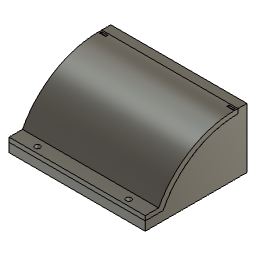
fanSocket (Autodesk Fusion 360 design; units mm, degrees)
Autodesk Fusion 360 part; units mm, degrees
sketch "Skizze1" plane through (0, 0, 0) normal (0, 1, 0) x (1, 0, 0)
  line L0 (0, 0) -> (40, 0)
  line L1 (40, 0) -> (40, -40)
  line L2 (40, -40) -> (0, -40)
  line L3 (0, -40) -> (0, 0)
  line L4 (4, -36) -> (36, -36) construction
  line L5 (36, -36) -> (36, -4) construction
  line L6 (36, -4) -> (4, -4) construction
  line L7 (4, -4) -> (4, -36) construction
  circle A0 centre (4, -36) radius 2.15
  circle A1 centre (36, -36) radius 2.15
  circle A2 centre (36, -4) radius 2.15
  circle A3 centre (4, -4) radius 2.15
  circle A4 centre (20, -20) radius 18
  dimension "d1" = 40
  dimension "d2" = 4.3
  dimension "d3" = 32
  dimension "d4" = 4
  dimension "d5" = 4
  dimension "d6" = 20
  dimension "d7" = 20
  dimension "d8" = 36
  constraint horizontal L0
  constraint vertical L1
  constraint horizontal L2
  constraint vertical L3
  constraint coincident L0.start L3.end
  constraint equal L0 L3
  constraint horizontal L4
  constraint vertical L5
  constraint horizontal L6
  constraint vertical L7
  constraint coincident L4.start L7.end
  constraint coincident L4.end L5.start
  constraint coincident L5.end L6.start
  constraint coincident L6.end L7.start
  constraint equal A0 A3
  constraint equal A0 A1
  constraint equal A1 A2
  constraint equal L4 L7
  measures "d1" distance of L0.start L2.end
  measures "d2" diameter of A0
  measures "d3" distance of L4.start L6.end
  measures "d4" vertical distance of L2.end L4.start
  measures "d5" horizontal distance of L2.end L4.start
  measures "d6" horizontal distance of L2.end A4.centre
  measures "d7" vertical distance of L1.end A4.centre
  measures "d8" diameter of A4
extrude "Extrusion1" add sketch "Skizze1" along normal blind 10 makes body 1
fillet "Abrundung1" radius 4 4 edges at (40, 5, 40) (40, 5, 0) (0, 5, 0) (0, 5, 40) on bodies 1
copy_body "Körper kopieren/einfügen1" bodies 1 makes body 2
move_body "Verschieben1" bodies 2 to x (1, 0, 0) y (0, 1, 0) z (0, 0, 1) at (41, 0, 0)
sketch "Skizze3" plane through (0, 0, 0) normal (0, 0, 1) x (1, 0, 0)
  line L0 (0, 0) -> (81, 0)
  line L1 (81, 0) -> (81, -55)
  line L2 (81, -55) -> (0, -55)
  line L3 (0, -55) -> (0, 0)
  circle A0 centre (20, -35) radius 18
  circle A1 centre (61, -35) radius 18
  circle A2 centre (40.5, -20) radius 2
  circle A3 centre (4, -51) radius 2
  circle A4 centre (77, -51) radius 2
  dimension "d15" = 20
  dimension "d16" = 20
  dimension "d17" = 36
  dimension "d18" = 40.5
  dimension "d19" = 20
  dimension "d20" = 4
  dimension "d21" = 4
  dimension "d22" = 4
  dimension "d23" = 4
  dimension "d24" = 4
  dimension "d25" = 81
  dimension "d26" = 35
  dimension "d27" = 35
  dimension "d28" = 55
  constraint horizontal L0
  constraint vertical L1
  constraint horizontal L2
  constraint vertical L3
  constraint coincident L0.start L3.end
  constraint equal A0 A1
  constraint equal A2 A3
  constraint equal A3 A4
  measures "d15" horizontal distance of L2.end A0.centre
  measures "d16" horizontal distance of L1.end A1.centre
  measures "d17" diameter of A0
  measures "d18" horizontal distance of L0.start A2.centre
  measures "d19" vertical distance of L0.start A2.centre
  measures "d20" vertical distance of L2.end A3.centre
  measures "d21" horizontal distance of L2.end A3.centre
  measures "d22" vertical distance of L1.end A4.centre
  measures "d23" horizontal distance of L1.end A4.centre
  measures "d24" diameter of A3
  measures "d25" distance of L0.start L0.end
  measures "d26" vertical distance of L0.start A0.centre
  measures "d27" vertical distance of L0.end A1.centre
  measures "d28" distance of L0.start L2.end
extrude "Extrusion2" add sketch "Skizze3" along normal blind 3 separate body makes body 3
move_body "Verschieben2" bodies 3 to x (1, 0, 0) y (0, 1, 0) z (0, 0, 1) at (0, -1, 0)
sketch "Skizze4" plane through (0, 0, 3) normal (0, 0, 1) x (-1, 0, 0)
  circle A0 centre (-40.5, 21) radius 2
  circle A1 centre (-61, 36) radius 18
  circle A2 centre (-20, 36) radius 18
  circle A3 centre (-4, 52) radius 2
  circle A4 centre (-77, 52) radius 2
  line L0 (0, 56) -> (-81, 56)
  line L1 (-81, 56) -> (-81, 1)
  line L2 (-81, 1) -> (0, 1)
  line L3 (0, 1) -> (0, 56)
  line L4 (0, 6) -> (-81, 6)
  dimension "d31" = 5
  constraint coincident L3 L4.start
  constraint coincident L1 L4.end
  constraint perpendicular L1 L4
  measures "d31" distance of L2.end L4.start
extrude "Extrusion3" add sketch "Skizze4" along normal blind 37 contours L1 L2 L3 L4 bodies 3
sketch "Skizze5" plane through (0, -6, 0) normal (0, -1, 0) x (1, 0, 0)
  line L0 (0, 3) -> (81, 3)
  line L1 (81, 3) -> (81, 40)
  line L2 (81, 40) -> (0, 40)
  line L3 (0, 40) -> (0, 3)
  line L4 (0, 20) -> (81, 20) construction
  circle A0 centre (20, 20) radius 18
  circle A1 centre (61, 20) radius 18
  line L5 (4, 36) -> (77, 36) construction
  line L6 (77, 36) -> (77, 4) construction
  line L7 (77, 4) -> (4, 4) construction
  line L8 (4, 4) -> (4, 36) construction
  circle A2 centre (4, 36) radius 2
  circle A3 centre (77, 36) radius 2
  circle A4 centre (77, 4) radius 2
  circle A5 centre (4, 4) radius 2
  line L9 (36, 36) -> (36, 4) construction
  line L10 (45, 4) -> (45, 36) construction
  circle A6 centre (36, 36) radius 2
  circle A7 centre (45, 36) radius 2
  circle A8 centre (45, 4) radius 2
  circle A9 centre (36, 4) radius 2
  dimension "d34" = 20
  dimension "d35" = 20
  dimension "d36" = 20
  dimension "d37" = 36
  dimension "d38" = 4
  dimension "d39" = 4
  dimension "d40" = 4
  dimension "d42" = 4
  dimension "d43" = 32
  dimension "d44" = 32
  dimension "d47" = 32
  constraint coincident L3 L4.start
  constraint coincident L1 L4.end
  constraint perpendicular L1 L4
  constraint coincident L4 A0.centre
  constraint coincident L4 A1.centre
  constraint equal A0 A1
  constraint perpendicular L1 L5
  constraint perpendicular L5 L8
  constraint vertical L6
  constraint horizontal L7
  constraint coincident L5.start L8.end
  constraint coincident L5.end L6.start
  constraint coincident L6.end L7.start
  constraint coincident L7.end L8.start
  constraint equal A2 A5
  constraint equal A2 A3
  constraint equal A3 A4
  constraint coincident L5 L9.start
  constraint coincident L7 L9.end
  constraint perpendicular L7 L9
  constraint coincident L7 L10.start
  constraint coincident L5 L10.end
  constraint perpendicular L5 L10
  constraint coincident L9.start A6.centre
  constraint coincident L10.end A7.centre
  constraint coincident L10.start A8.centre
  constraint coincident L9.end A9.centre
  constraint equal A8 A9
  constraint equal A7 A8
  constraint equal A6 A7
  constraint equal A2 A6
  measures "d34" distance of L2.end L4.start
  measures "d35" distance of L4.start A0.centre
  measures "d36" horizontal distance of L1.end A1.centre
  measures "d37" diameter of A0
  measures "d38" horizontal distance of L2.end L5.start
  measures "d39" vertical distance of L2.end L5.start
  measures "d40" horizontal distance of L1.end L5.end
  measures "d42" diameter of A2
  measures "d43" distance of L5.end L10.end
  measures "d44" distance of L5.start L9.start
  measures "d47" distance of L5.end L6.end
extrude "Extrusion4" cut sketch "Skizze5" against normal blind 10 contours L0 A5 | L0 A5 | L0 A0 | L0 A0 | L0 A4 | L0 A4 | L0 A9 | L0 A9 | L0 A1 | L0 A1 | L0 A8 | L0 A8 | A2 | A3 | A6 | A7 bodies 3
extrude "Extrusion18" add 1 faces at (0, -2.6667, 14.3333) along direction (-1, 0, 0) blind 5 on bodies 3 bodies 3
extrude "Extrusion19" add 1 faces at (81, -2.6667, 14.3333) along direction (1, 0, 0) blind 5 on bodies 3 bodies 3
sketch "Skizze14" plane through (0, 0, 3) normal (0, 0, 1) x (-1, 0, 0)
  circle A0 centre (-61, 36) radius 18
  circle A1 centre (-20, 36) radius 18
  circle A2 centre (-77, 52) radius 2
  circle A3 centre (-40.5, 21) radius 2
  circle A4 centre (-4, 52) radius 2
  line L0 (-75.2679, 6) -> (-66.9161, 6)
  line L1 (5, 6) -> (5, 56)
  line L2 (5, 56) -> (-86, 56)
  line L3 (-86, 56) -> (-86, 6)
  line L4 (-86, 6) -> (-78.7321, 6)
  line L5 (-25.4828, 18.8553) -> (-37.1447, 30.5172)
  line L6 (-21.8995, 18.1005) -> (-37.8995, 34.1005)
  line L7 (-17.7035, 18.1471) -> (-37.8529, 38.2965)
  line L8 (-15.3413, 18.6133) -> (-37.3867, 40.6587)
  line L9 (-12.2426, 19.7574) -> (-36.2426, 43.7574)
  line L10 (-10.4188, 20.7619) -> (-35.2381, 45.5812)
  line L11 (-7.9988, 22.5846) -> (-33.4154, 48.0012)
  line L12 (-6.5846, 23.9988) -> (-32.0012, 49.4154)
  line L13 (-4.7619, 26.4188) -> (-29.5812, 51.2381)
  line L14 (-3.7574, 28.2426) -> (-27.7574, 52.2426)
  line L15 (-2.6133, 31.3413) -> (-24.6587, 53.3867)
  line L16 (-2.1471, 33.7035) -> (-22.2965, 53.8529)
  line L17 (-2.1005, 37.8995) -> (-18.1005, 53.8995)
  line L18 (-2.8553, 41.4828) -> (-14.5172, 53.1447)
  line L19 (-66.4828, 18.8553) -> (-78.1447, 30.5172)
  line L20 (-62.8995, 18.1005) -> (-78.8995, 34.1005)
  line L21 (-58.7035, 18.1471) -> (-78.8529, 38.2965)
  line L22 (-56.3413, 18.6133) -> (-78.3867, 40.6587)
  line L23 (-53.2426, 19.7574) -> (-77.2426, 43.7574)
  line L24 (-51.4188, 20.7619) -> (-76.2381, 45.5812)
  line L25 (-48.9988, 22.5846) -> (-74.4154, 48.0012)
  line L26 (-47.5846, 23.9988) -> (-73.0012, 49.4154)
  line L27 (-45.7619, 26.4188) -> (-70.5812, 51.2381)
  line L28 (-44.7574, 28.2426) -> (-68.7574, 52.2426)
  line L29 (-43.6133, 31.3413) -> (-65.6587, 53.3867)
  line L30 (-43.1471, 33.7035) -> (-63.2965, 53.8529)
  line L31 (-59.1005, 53.8995) -> (-43.1005, 37.8995)
  line L32 (-43.8553, 41.4828) -> (-55.5172, 53.1447)
  line L33 (-78.7321, 6) -> (-75.2679, 6)
  line L34 (-66.9161, 6) -> (-55.0839, 6)
  line L35 (-55.0839, 6) -> (-46.7321, 6)
  line L36 (-46.7321, 6) -> (-43.2679, 6)
  line L37 (-43.2679, 6) -> (-37.7321, 6)
  line L38 (-37.7321, 6) -> (-34.2679, 6)
  line L39 (-34.2679, 6) -> (-25.9161, 6)
  line L40 (-25.9161, 6) -> (-14.0839, 6)
  line L41 (-14.0839, 6) -> (-5.7321, 6)
  line L42 (-5.7321, 6) -> (-2.2679, 6)
  line L43 (-2.2679, 6) -> (5, 6)
  dimension "d107" = 2
  dimension "d108" = 3
  dimension "d109" = 2
  dimension "d110" = 3
  dimension "d111" = 2
  dimension "d112" = 3
  dimension "d113" = 2
  dimension "d114" = 16
  dimension "d126" = 3
  dimension "d127" = 2
  dimension "d128" = 3
  dimension "d131" = 2
  dimension "d132" = 3
  dimension "d136" = 2
  dimension "d137" = 16
  dimension "d138" = 2
  dimension "d139" = 3
  dimension "d140" = 2
  dimension "d141" = 3
  dimension "d142" = 2
  dimension "d143" = 3
  dimension "d144" = 2
  dimension "d145" = 3
  dimension "d146" = 2
  dimension "d147" = 3
  dimension "d148" = 2
  dimension "d149" = 3
  dimension "d150" = 2
  constraint coincident A1 L5.start
  constraint coincident A1 L5.end
  constraint coincident A1 L6.start
  constraint coincident A1 L6.end
  constraint coincident A1 L7.start
  constraint coincident A1 L7.end
  constraint coincident A1 L8.start
  constraint coincident A1 L8.end
  constraint coincident A1 L9.start
  constraint coincident A1 L9.end
  constraint coincident A1 L10.start
  constraint coincident A1 L10.end
  constraint coincident A1 L11.start
  constraint coincident A1 L11.end
  constraint coincident A1 L12.start
  constraint coincident A1 L12.end
  constraint parallel L5 L6
  constraint parallel L6 L7
  constraint parallel L7 L8
  constraint parallel L8 L9
  constraint parallel L9 L10
  constraint parallel L10 L11
  constraint parallel L11 L12
  constraint coincident A1 L13.start
  constraint coincident A1 L13.end
  constraint coincident A1 L14.start
  constraint coincident A1 L14.end
  constraint coincident A1 L15.start
  constraint coincident A1 L15.end
  constraint parallel L12 L13
  constraint parallel L13 L14
  constraint parallel L14 L15
  constraint coincident A1 L16.start
  constraint coincident A1 L16.end
  constraint coincident A1 L17.start
  constraint coincident A1 L17.end
  constraint parallel L15 L16
  constraint parallel L15 L17
  constraint coincident A1 L18.start
  constraint coincident A1 L18.end
  constraint parallel L17 L18
  constraint coincident A0 L19.start
  constraint coincident A0 L19.end
  constraint coincident A0 L20.start
  constraint coincident A0 L20.end
  constraint coincident A0 L21.start
  constraint coincident A0 L21.end
  constraint coincident A0 L22.start
  constraint coincident A0 L22.end
  constraint coincident A0 L23.start
  constraint coincident A0 L23.end
  constraint coincident A0 L24.start
  constraint coincident A0 L24.end
  constraint coincident A0 L25.start
  constraint coincident A0 L25.end
  constraint coincident A0 L26.start
  constraint coincident A0 L26.end
  constraint coincident A0 L27.start
  constraint coincident A0 L27.end
  constraint coincident A0 L28.start
  constraint coincident A0 L28.end
  constraint coincident A0 L29.start
  constraint coincident A0 L29.end
  constraint coincident A0 L30.start
  constraint coincident A0 L30.end
  constraint coincident A0 L31.start
  constraint coincident A0 L31.end
  constraint coincident A0 L32.start
  constraint coincident A0 L32.end
  constraint parallel L19 L20
  constraint parallel L20 L21
  constraint parallel L21 L22
  constraint parallel L22 L23
  constraint parallel L23 L24
  constraint parallel L24 L25
  constraint parallel L25 L26
  constraint parallel L26 L27
  constraint parallel L27 L28
  constraint parallel L28 L29
  constraint parallel L29 L30
  constraint parallel L30 L31
  constraint parallel L31 L32
  measures "d107" distance of L5 L6
  measures "d108" distance of L6 L7
  measures "d109" distance of L7 L8
  measures "d110" distance of L8 L9
  measures "d111" distance of L9 L10
  measures "d112" distance of L10 L11
  measures "d113" distance of L11 L12
  measures "d114" distance of A1.centre L5
  measures "d126" distance of L12 L13
  measures "d127" distance of L13 L14
  measures "d128" distance of L14 L15
  measures "d131" distance of L15 L16
  measures "d132" distance of L16 L17
  measures "d136" distance of L17 L18
  measures "d137" distance of A0.centre L19
  measures "d138" distance of L19 L20
  measures "d139" distance of L20 L21
  measures "d140" distance of L21 L22
  measures "d141" distance of L22 L23
  measures "d142" distance of L23 L24
  measures "d143" distance of L24 L25
  measures "d144" distance of L25 L26
  measures "d145" distance of L26 L27
  measures "d146" distance of L27 L28
  measures "d147" distance of L28 L29
  measures "d148" distance of L29 L30
  measures "d149" distance of L30 L31
  measures "d150" distance of L31 L32
extrude "Extrusion25" add sketch "Skizze14" against normal blind 3 contours A0 L31 L32 | A0 L29 L30 | A0 L27 L28 | A0 L25 L26 | A0 L23 L24 | A0 L21 L22 | A0 L19 L20 | A1 L17 L18 | A1 L15 L16 | A1 L13 L14 | A1 L11 L12 | A1 L9 L10 | A1 L7 L8 | A1 L5 L6 bodies 3
extrude "Extrusion28" add 1 faces at (25.3333, -56, 1) along direction (0, -1, 0) blind 12 on bodies 3 bodies 3
sketch "Skizze19" plane through (0, 0, 3) normal (0, 0, 1) x (-1, 0, 0)
  circle A0 centre (-40.5, 21) radius 2
  circle A1 centre (-4, 52) radius 2
  circle A2 centre (-77, 52) radius 2
  line L0 (-78.1447, 30.5172) -> (-66.4828, 18.8553)
  arc A3 (-78.1447, 30.5172) -> (-66.4828, 18.8553) centre (-61, 36) ccw
  line L1 (-37.1447, 30.5172) -> (-25.4828, 18.8553)
  arc A4 (-37.1447, 30.5172) -> (-25.4828, 18.8553) centre (-20, 36) ccw
  line L2 (-74.4154, 48.0012) -> (-48.9988, 22.5846)
  arc A5 (-51.4188, 20.7619) -> (-48.9988, 22.5846) centre (-61, 36) ccw
  line L3 (-51.4188, 20.7619) -> (-76.2381, 45.5812)
  arc A6 (-74.4154, 48.0012) -> (-76.2381, 45.5812) centre (-61, 36) ccw
  arc A7 (-43.8553, 41.4828) -> (-55.5172, 53.1447) centre (-61, 36) ccw
  line L4 (-43.8553, 41.4828) -> (-55.5172, 53.1447)
  line L5 (-29.5812, 51.2381) -> (-4.7619, 26.4188)
  arc A8 (-6.5846, 23.9988) -> (-4.7619, 26.4188) centre (-20, 36) ccw
  line L6 (-6.5846, 23.9988) -> (-32.0012, 49.4154)
  arc A9 (-29.5812, 51.2381) -> (-32.0012, 49.4154) centre (-20, 36) ccw
  line L7 (-37.8529, 38.2965) -> (-17.7035, 18.1471)
  arc A10 (-21.8995, 18.1005) -> (-17.7035, 18.1471) centre (-20, 36) ccw
  line L8 (-21.8995, 18.1005) -> (-37.8995, 34.1005)
  arc A11 (-37.8529, 38.2965) -> (-37.8995, 34.1005) centre (-20, 36) ccw
  line L9 (-24.6587, 53.3867) -> (-2.6133, 31.3413)
  arc A12 (-3.7574, 28.2426) -> (-2.6133, 31.3413) centre (-20, 36) ccw
  line L10 (-3.7574, 28.2426) -> (-27.7574, 52.2426)
  arc A13 (-24.6587, 53.3867) -> (-27.7574, 52.2426) centre (-20, 36) ccw
  arc A14 (-59.1005, 53.8995) -> (-63.2965, 53.8529) centre (-61, 36) ccw
  line L11 (-59.1005, 53.8995) -> (-43.1005, 37.8995)
  arc A15 (-43.1471, 33.7035) -> (-43.1005, 37.8995) centre (-61, 36) ccw
  line L12 (-43.1471, 33.7035) -> (-63.2965, 53.8529)
  arc A16 (-77.2426, 43.7574) -> (-78.3867, 40.6587) centre (-61, 36) ccw
  line L13 (-77.2426, 43.7574) -> (-53.2426, 19.7574)
  arc A17 (-56.3413, 18.6133) -> (-53.2426, 19.7574) centre (-61, 36) ccw
  line L14 (-56.3413, 18.6133) -> (-78.3867, 40.6587)
  line L15 (-70.5812, 51.2381) -> (-45.7619, 26.4188)
  arc A18 (-47.5846, 23.9988) -> (-45.7619, 26.4188) centre (-61, 36) ccw
  line L16 (-47.5846, 23.9988) -> (-73.0012, 49.4154)
  arc A19 (-70.5812, 51.2381) -> (-73.0012, 49.4154) centre (-61, 36) ccw
  arc A20 (-2.8553, 41.4828) -> (-14.5172, 53.1447) centre (-20, 36) ccw
  line L17 (-2.8553, 41.4828) -> (-14.5172, 53.1447)
  arc A21 (-33.4154, 48.0012) -> (-35.2381, 45.5812) centre (-20, 36) ccw
  line L18 (-33.4154, 48.0012) -> (-7.9988, 22.5846)
  arc A22 (-10.4188, 20.7619) -> (-7.9988, 22.5846) centre (-20, 36) ccw
  line L19 (-10.4188, 20.7619) -> (-35.2381, 45.5812)
  arc A23 (-36.2426, 43.7574) -> (-37.3867, 40.6587) centre (-20, 36) ccw
  line L20 (-36.2426, 43.7574) -> (-12.2426, 19.7574)
  arc A24 (-15.3413, 18.6133) -> (-12.2426, 19.7574) centre (-20, 36) ccw
  line L21 (-15.3413, 18.6133) -> (-37.3867, 40.6587)
  arc A25 (-18.1005, 53.8995) -> (-22.2965, 53.8529) centre (-20, 36) ccw
  line L22 (-18.1005, 53.8995) -> (-2.1005, 37.8995)
  arc A26 (-2.1471, 33.7035) -> (-2.1005, 37.8995) centre (-20, 36) ccw
  line L23 (-2.1471, 33.7035) -> (-22.2965, 53.8529)
  arc A27 (-65.6587, 53.3867) -> (-68.7574, 52.2426) centre (-61, 36) ccw
  line L24 (-65.6587, 53.3867) -> (-43.6133, 31.3413)
  arc A28 (-44.7574, 28.2426) -> (-43.6133, 31.3413) centre (-61, 36) ccw
  line L25 (-44.7574, 28.2426) -> (-68.7574, 52.2426)
  arc A29 (-78.8529, 38.2965) -> (-78.8995, 34.1005) centre (-61, 36) ccw
  line L26 (-78.8529, 38.2965) -> (-58.7035, 18.1471)
  arc A30 (-62.8995, 18.1005) -> (-58.7035, 18.1471) centre (-61, 36) ccw
  line L27 (-62.8995, 18.1005) -> (-78.8995, 34.1005)
  line L28 (-86, 6) -> (-78.7321, 6)
  line L29 (5, 6) -> (5, 68)
  line L30 (5, 68) -> (-86, 68)
  line L31 (-86, 68) -> (-86, 6)
  line L32 (5, 64) -> (-86, 64) construction
  circle A31 centre (-10, 64) radius 2
  circle A32 centre (-71, 64) radius 2
  line L33 (-78.7321, 6) -> (-75.2679, 6)
  line L34 (-75.2679, 6) -> (-66.9161, 6)
  line L35 (-66.9161, 6) -> (-55.0839, 6)
  line L36 (-55.0839, 6) -> (-46.7321, 6)
  line L37 (-46.7321, 6) -> (-43.2679, 6)
  line L38 (-43.2679, 6) -> (-37.7321, 6)
  line L39 (-37.7321, 6) -> (-34.2679, 6)
  line L40 (-34.2679, 6) -> (-25.9161, 6)
  line L41 (-25.9161, 6) -> (-14.0839, 6)
  line L42 (-14.0839, 6) -> (-5.7321, 6)
  line L43 (-5.7321, 6) -> (-2.2679, 6)
  line L44 (-2.2679, 6) -> (5, 6)
  dimension "d163" = 4
  dimension "d164" = 15
  dimension "d165" = 15
  dimension "d176" = 4
  dimension "d177" = 91
  constraint coincident L32 A31.centre
  constraint coincident L32 A32.centre
  constraint equal A31 A32
  constraint horizontal L32
  constraint coincident L29 L32.start
  measures "d163" diameter of A31
  measures "d164" distance of L32.start A31.centre
  measures "d165" distance of L32.end A32.centre
  measures "d176" distance of L29.end L32.start
  measures "d177" distance of L32.start L32.end
extrude "Extrusion29" cut sketch "Skizze19" against normal blind 5 contours A31 | A32 bodies 3
sketch "Skizze21" plane through (0, 0, 3) normal (0, 0, 1) x (-1, 0, 0)
  circle A0 centre (-40.5, 21) radius 2
  circle A1 centre (-4, 52) radius 2
  circle A2 centre (-77, 52) radius 2
  line L0 (-78.1447, 30.5172) -> (-66.4828, 18.8553)
  arc A3 (-78.1447, 30.5172) -> (-66.4828, 18.8553) centre (-61, 36) ccw
  line L1 (-37.1447, 30.5172) -> (-25.4828, 18.8553)
  arc A4 (-37.1447, 30.5172) -> (-25.4828, 18.8553) centre (-20, 36) ccw
  line L2 (-74.4154, 48.0012) -> (-48.9988, 22.5846)
  arc A5 (-51.4188, 20.7619) -> (-48.9988, 22.5846) centre (-61, 36) ccw
  line L3 (-51.4188, 20.7619) -> (-76.2381, 45.5812)
  arc A6 (-74.4154, 48.0012) -> (-76.2381, 45.5812) centre (-61, 36) ccw
  arc A7 (-43.8553, 41.4828) -> (-55.5172, 53.1447) centre (-61, 36) ccw
  line L4 (-43.8553, 41.4828) -> (-55.5172, 53.1447)
  line L5 (-29.5812, 51.2381) -> (-4.7619, 26.4188)
  arc A8 (-6.5846, 23.9988) -> (-4.7619, 26.4188) centre (-20, 36) ccw
  line L6 (-6.5846, 23.9988) -> (-32.0012, 49.4154)
  arc A9 (-29.5812, 51.2381) -> (-32.0012, 49.4154) centre (-20, 36) ccw
  line L7 (-37.8529, 38.2965) -> (-17.7035, 18.1471)
  arc A10 (-21.8995, 18.1005) -> (-17.7035, 18.1471) centre (-20, 36) ccw
  line L8 (-21.8995, 18.1005) -> (-37.8995, 34.1005)
  arc A11 (-37.8529, 38.2965) -> (-37.8995, 34.1005) centre (-20, 36) ccw
  line L9 (-24.6587, 53.3867) -> (-2.6133, 31.3413)
  arc A12 (-3.7574, 28.2426) -> (-2.6133, 31.3413) centre (-20, 36) ccw
  line L10 (-3.7574, 28.2426) -> (-27.7574, 52.2426)
  arc A13 (-24.6587, 53.3867) -> (-27.7574, 52.2426) centre (-20, 36) ccw
  arc A14 (-59.1005, 53.8995) -> (-63.2965, 53.8529) centre (-61, 36) ccw
  line L11 (-59.1005, 53.8995) -> (-43.1005, 37.8995)
  arc A15 (-43.1471, 33.7035) -> (-43.1005, 37.8995) centre (-61, 36) ccw
  line L12 (-43.1471, 33.7035) -> (-63.2965, 53.8529)
  arc A16 (-77.2426, 43.7574) -> (-78.3867, 40.6587) centre (-61, 36) ccw
  line L13 (-77.2426, 43.7574) -> (-53.2426, 19.7574)
  arc A17 (-56.3413, 18.6133) -> (-53.2426, 19.7574) centre (-61, 36) ccw
  line L14 (-56.3413, 18.6133) -> (-78.3867, 40.6587)
  line L15 (-70.5812, 51.2381) -> (-45.7619, 26.4188)
  arc A18 (-47.5846, 23.9988) -> (-45.7619, 26.4188) centre (-61, 36) ccw
  line L16 (-47.5846, 23.9988) -> (-73.0012, 49.4154)
  arc A19 (-70.5812, 51.2381) -> (-73.0012, 49.4154) centre (-61, 36) ccw
  arc A20 (-2.8553, 41.4828) -> (-14.5172, 53.1447) centre (-20, 36) ccw
  line L17 (-2.8553, 41.4828) -> (-14.5172, 53.1447)
  arc A21 (-33.4154, 48.0012) -> (-35.2381, 45.5812) centre (-20, 36) ccw
  line L18 (-33.4154, 48.0012) -> (-7.9988, 22.5846)
  arc A22 (-10.4188, 20.7619) -> (-7.9988, 22.5846) centre (-20, 36) ccw
  line L19 (-10.4188, 20.7619) -> (-35.2381, 45.5812)
  arc A23 (-36.2426, 43.7574) -> (-37.3867, 40.6587) centre (-20, 36) ccw
  line L20 (-36.2426, 43.7574) -> (-12.2426, 19.7574)
  arc A24 (-15.3413, 18.6133) -> (-12.2426, 19.7574) centre (-20, 36) ccw
  line L21 (-15.3413, 18.6133) -> (-37.3867, 40.6587)
  arc A25 (-18.1005, 53.8995) -> (-22.2965, 53.8529) centre (-20, 36) ccw
  line L22 (-18.1005, 53.8995) -> (-2.1005, 37.8995)
  arc A26 (-2.1471, 33.7035) -> (-2.1005, 37.8995) centre (-20, 36) ccw
  line L23 (-2.1471, 33.7035) -> (-22.2965, 53.8529)
  arc A27 (-65.6587, 53.3867) -> (-68.7574, 52.2426) centre (-61, 36) ccw
  line L24 (-65.6587, 53.3867) -> (-43.6133, 31.3413)
  arc A28 (-44.7574, 28.2426) -> (-43.6133, 31.3413) centre (-61, 36) ccw
  line L25 (-44.7574, 28.2426) -> (-68.7574, 52.2426)
  arc A29 (-78.8529, 38.2965) -> (-78.8995, 34.1005) centre (-61, 36) ccw
  line L26 (-78.8529, 38.2965) -> (-58.7035, 18.1471)
  arc A30 (-62.8995, 18.1005) -> (-58.7035, 18.1471) centre (-61, 36) ccw
  line L27 (-62.8995, 18.1005) -> (-78.8995, 34.1005)
  line L28 (-86, 6) -> (-78.7321, 6)
  line L29 (5, 6) -> (5, 68)
  line L30 (5, 68) -> (-86, 68)
  line L31 (-86, 68) -> (-86, 6)
  line L32 (5, 56) -> (-86, 56)
  circle A31 centre (-71, 64) radius 2
  circle A32 centre (-10, 64) radius 2
  line L33 (-78.7321, 6) -> (-75.2679, 6)
  line L34 (-75.2679, 6) -> (-66.9161, 6)
  line L35 (-66.9161, 6) -> (-55.0839, 6)
  line L36 (-55.0839, 6) -> (-46.7321, 6)
  line L37 (-46.7321, 6) -> (-43.2679, 6)
  line L38 (-43.2679, 6) -> (-37.7321, 6)
  line L39 (-37.7321, 6) -> (-34.2679, 6)
  line L40 (-34.2679, 6) -> (-25.9161, 6)
  line L41 (-25.9161, 6) -> (-14.0839, 6)
  line L42 (-14.0839, 6) -> (-5.7321, 6)
  line L43 (-5.7321, 6) -> (-2.2679, 6)
  line L44 (-2.2679, 6) -> (5, 6)
  dimension "d172" = 12
  constraint coincident L29 L32.start
  constraint coincident L31 L32.end
  constraint perpendicular L31 L32
  measures "d172" distance of L29.end L32.start
extrude "Extrusion32" add sketch "Skizze21" along normal blind 3 contours L29 L30 L31 L32 bodies 3
sketch "Skizze22" plane through (-5, 0, 0) normal (-1, 0, 0) x (0, -1, 0)
  line L0 (1, 0) -> (68, 0)
  line L1 (68, 0) -> (68, 6)
  line L2 (68, 6) -> (56, 6)
  line L3 (56, 6) -> (56, 3)
  line L4 (56, 3) -> (6, 3)
  line L5 (6, 3) -> (6, 40)
  line L6 (6, 40) -> (1, 40)
  line L7 (1, 40) -> (1, 0)
  arc A0 (56, 6) -> (6, 37) centre (6, -18.8226) ccw
  line L8 (6, 37) -> (1, 37)
  dimension "d182" = 3
  constraint coincident L2.end L3.start
  constraint coincident L5 A0.end
  constraint coincident L7 L8.end
  constraint perpendicular L7 L8
  constraint tangent A0 L8
  measures "d182" distance of L5.end A0.end
extrude "Extrusion34" add sketch "Skizze22" against normal blind 3 contours L3 L4 L5 A0 bodies 3
sketch "Skizze23" plane through (86, 0, 0) normal (1, 0, 0) x (0, 1, 0)
  line L0 (-68, 0) -> (-1, 0)
  line L1 (-1, 0) -> (-1, 40)
  line L2 (-1, 40) -> (-6, 40)
  line L3 (-6, 40) -> (-6, 3)
  line L4 (-6, 3) -> (-56, 3)
  line L5 (-56, 3) -> (-56, 6)
  line L6 (-56, 6) -> (-68, 6)
  line L7 (-68, 6) -> (-68, 0)
  arc A0 (-6, 37) -> (-56, 6) centre (-6, -18.8226) ccw
  line L8 (-6, 37) -> (-1, 37)
  dimension "d185" = 3
  constraint coincident L5.end L6.start
  constraint coincident L3 A0.start
  constraint coincident L1 L8.end
  constraint tangent A0 L8
  constraint horizontal L8
  measures "d185" distance of L2.end A0.start
extrude "Extrusion35" add sketch "Skizze23" against normal blind 3 contours L3 L4 L5 A0 bodies 3
sketch "Skizze24" plane through (0, 0, 0) normal (1, 0, 0) x (0, 1, 0)
  arc A0 (-6, 37) -> (-56, 6) centre (-6.2378, -18.439) ccw
  line L0 (-6, 37) -> (-6, 40)
  line L1 (-56, 6) -> (-59, 6)
  line L2 (-59, 6) -> (-59, 9) construction
  arc A1 (-6, 40) -> (-59, 9) centre (-7.9795, -17.4222) ccw
  line L3 (-59, 9) -> (-68, 9)
  line L4 (-68, 9) -> (-68, 6)
  line L5 (-68, 6) -> (-59, 6)
  dimension "d188" = 3
  dimension "d189" = 9
  dimension "d190" = 3
  constraint vertical L0
  constraint horizontal L1
  constraint perpendicular L1 L2
  constraint tangent A0 A1
  constraint perpendicular L2 L3
  constraint perpendicular L3 L4
  constraint perpendicular L2 L5
  measures "d188" distance of A0.end L1.end
  measures "d189" distance of L2.end L3.end
  measures "d190" distance of L3.end L4.end
extrude "Extrusion36" add sketch "Skizze24" along normal blind 91 separate body makes body 4
move_body "Verschieben4" bodies 4 to x (1, 0, 0) y (0, 1, 0) z (0, 0, 1) at (-5, 0, 0)
sketch "Skizze26" plane through (0, 0, 6) normal (0, 0, -1) x (1, 0, 0)
  line L0 (-5, 68) -> (-5, 59)
  line L1 (-5, 59) -> (86, 59)
  line L2 (86, 59) -> (86, 68)
  line L3 (86, 68) -> (-5, 68)
  circle A0 centre (10, 64) radius 1.75
  circle A1 centre (71, 64) radius 1.75
  dimension "d193" = 3.5
  dimension "d194" = 3.5
  measures "d193" diameter of A1
  measures "d194" diameter of A0
extrude "Extrusion37" cut sketch "Skizze26" against normal blind 10 contours A0 | A1 bodies 4
sketch "Skizze30" plane through (0, -6, 0) normal (0, -1, 0) x (1, 0, 0)
  line L0 (83, 37) -> (86, 37)
  line L1 (86, 37) -> (86, 40)
  line L2 (86, 40) -> (-5, 40)
  line L3 (-5, 40) -> (-5, 37)
  line L4 (-5, 37) -> (-2, 37)
  line L5 (-2, 37) -> (-2, 3)
  line L6 (-2, 3) -> (2.2679, 3)
  line L7 (78.7321, 3) -> (83, 3)
  line L8 (83, 3) -> (83, 37)
  circle A0 centre (77, 36) radius 2
  circle A1 centre (4, 36) radius 2
  circle A2 centre (36, 36) radius 2
  circle A3 centre (45, 36) radius 2
  arc A4 (5.7321, 3) -> (2.2679, 3) centre (4, 4) ccw
  line L9 (5.7321, 3) -> (14.0839, 3)
  arc A5 (25.9161, 3) -> (14.0839, 3) centre (20, 20) ccw
  line L10 (25.9161, 3) -> (34.2679, 3)
  arc A6 (37.7321, 3) -> (34.2679, 3) centre (36, 4) ccw
  line L11 (37.7321, 3) -> (43.2679, 3)
  arc A7 (46.7321, 3) -> (43.2679, 3) centre (45, 4) ccw
  line L12 (46.7321, 3) -> (55.0839, 3)
  arc A8 (66.9161, 3) -> (55.0839, 3) centre (61, 20) ccw
  line L13 (66.9161, 3) -> (75.2679, 3)
  arc A9 (78.7321, 3) -> (75.2679, 3) centre (77, 4) ccw
  line L14 (-4, 38.5) -> (0, 38.5)
  line L15 (0, 38.5) -> (0, 37)
  line L16 (0, 37) -> (-4, 37)
  line L17 (-4, 37) -> (-4, 38.5)
  line L18 (85, 38.5) -> (81, 38.5)
  line L19 (81, 38.5) -> (81, 37)
  line L20 (81, 37) -> (85, 37)
  line L21 (85, 37) -> (85, 38.5)
  dimension "d237" = 4
  dimension "d238" = 1.5
  dimension "d239" = 1.5
  dimension "d240" = 1
  dimension "d241" = 4
  dimension "d242" = 1.5
  dimension "d243" = 1
  dimension "d244" = 1.5
  constraint horizontal L14
  constraint vertical L15
  constraint horizontal L16
  constraint vertical L17
  constraint horizontal L18
  constraint vertical L19
  constraint horizontal L20
  constraint vertical L21
  measures "d237" distance of L14.start L14.end
  measures "d238" vertical distance of L2.end L14.start
  measures "d239" distance of L14.start L16.end
  measures "d240" horizontal distance of L2.end L14.start
  measures "d241" distance of L18.start L18.end
  measures "d242" vertical distance of L1.end L18.start
  measures "d243" horizontal distance of L1.end L18.start
  measures "d244" distance of L18.start L20.end
extrude "Extrusion41" add 1 faces at (83.6667, -1, 20) along direction (0, 1, 0) blind 1 on bodies 3 bodies 3
sketch "Skizze31" plane through (0, 0, 3) normal (0, 0, 1) x (-1, 0, 0)
  line L0 (-83, 56) -> (-83, 6)
  line L1 (-83, 6) -> (-78.7321, 6)
  line L2 (-78.7321, 6) -> (-75.2679, 6)
  line L3 (-75.2679, 6) -> (-66.9161, 6)
  line L4 (-66.9161, 6) -> (-55.0839, 6)
  line L5 (-55.0839, 6) -> (-46.7321, 6)
  line L6 (-46.7321, 6) -> (-43.2679, 6)
  line L7 (-43.2679, 6) -> (-37.7321, 6)
  line L8 (-37.7321, 6) -> (-34.2679, 6)
  line L9 (-34.2679, 6) -> (-25.9161, 6)
  line L10 (-25.9161, 6) -> (-14.0839, 6)
  line L11 (-14.0839, 6) -> (-5.7321, 6)
  line L12 (-5.7321, 6) -> (-2.2679, 6)
  line L13 (-2.2679, 6) -> (2, 6)
  line L14 (2, 6) -> (2, 56)
  line L15 (2, 56) -> (-83, 56)
  arc A0 (-78.8529, 38.2965) -> (-78.8995, 34.1005) centre (-61, 36) ccw
  line L16 (-78.8529, 38.2965) -> (-58.7035, 18.1471)
  arc A1 (-62.8995, 18.1005) -> (-58.7035, 18.1471) centre (-61, 36) ccw
  line L17 (-62.8995, 18.1005) -> (-78.8995, 34.1005)
  arc A2 (-65.6587, 53.3867) -> (-68.7574, 52.2426) centre (-61, 36) ccw
  line L18 (-65.6587, 53.3867) -> (-43.6133, 31.3413)
  arc A3 (-44.7574, 28.2426) -> (-43.6133, 31.3413) centre (-61, 36) ccw
  line L19 (-44.7574, 28.2426) -> (-68.7574, 52.2426)
  arc A4 (-18.1005, 53.8995) -> (-22.2965, 53.8529) centre (-20, 36) ccw
  line L20 (-18.1005, 53.8995) -> (-2.1005, 37.8995)
  arc A5 (-2.1471, 33.7035) -> (-2.1005, 37.8995) centre (-20, 36) ccw
  line L21 (-2.1471, 33.7035) -> (-22.2965, 53.8529)
  arc A6 (-36.2426, 43.7574) -> (-37.3867, 40.6587) centre (-20, 36) ccw
  line L22 (-36.2426, 43.7574) -> (-12.2426, 19.7574)
  arc A7 (-15.3413, 18.6133) -> (-12.2426, 19.7574) centre (-20, 36) ccw
  line L23 (-15.3413, 18.6133) -> (-37.3867, 40.6587)
  arc A8 (-33.4154, 48.0012) -> (-35.2381, 45.5812) centre (-20, 36) ccw
  line L24 (-33.4154, 48.0012) -> (-7.9988, 22.5846)
  arc A9 (-10.4188, 20.7619) -> (-7.9988, 22.5846) centre (-20, 36) ccw
  line L25 (-10.4188, 20.7619) -> (-35.2381, 45.5812)
  arc A10 (-2.8553, 41.4828) -> (-14.5172, 53.1447) centre (-20, 36) ccw
  line L26 (-2.8553, 41.4828) -> (-14.5172, 53.1447)
  line L27 (-70.5812, 51.2381) -> (-45.7619, 26.4188)
  arc A11 (-47.5846, 23.9988) -> (-45.7619, 26.4188) centre (-61, 36) ccw
  line L28 (-47.5846, 23.9988) -> (-73.0012, 49.4154)
  arc A12 (-70.5812, 51.2381) -> (-73.0012, 49.4154) centre (-61, 36) ccw
  arc A13 (-77.2426, 43.7574) -> (-78.3867, 40.6587) centre (-61, 36) ccw
  line L29 (-77.2426, 43.7574) -> (-53.2426, 19.7574)
  arc A14 (-56.3413, 18.6133) -> (-53.2426, 19.7574) centre (-61, 36) ccw
  line L30 (-56.3413, 18.6133) -> (-78.3867, 40.6587)
  arc A15 (-59.1005, 53.8995) -> (-63.2965, 53.8529) centre (-61, 36) ccw
  line L31 (-59.1005, 53.8995) -> (-43.1005, 37.8995)
  arc A16 (-43.1471, 33.7035) -> (-43.1005, 37.8995) centre (-61, 36) ccw
  line L32 (-43.1471, 33.7035) -> (-63.2965, 53.8529)
  line L33 (-24.6587, 53.3867) -> (-2.6133, 31.3413)
  arc A17 (-3.7574, 28.2426) -> (-2.6133, 31.3413) centre (-20, 36) ccw
  line L34 (-3.7574, 28.2426) -> (-27.7574, 52.2426)
  arc A18 (-24.6587, 53.3867) -> (-27.7574, 52.2426) centre (-20, 36) ccw
  line L35 (-37.8529, 38.2965) -> (-17.7035, 18.1471)
  arc A19 (-21.8995, 18.1005) -> (-17.7035, 18.1471) centre (-20, 36) ccw
  line L36 (-21.8995, 18.1005) -> (-37.8995, 34.1005)
  arc A20 (-37.8529, 38.2965) -> (-37.8995, 34.1005) centre (-20, 36) ccw
  line L37 (-29.5812, 51.2381) -> (-4.7619, 26.4188)
  arc A21 (-6.5846, 23.9988) -> (-4.7619, 26.4188) centre (-20, 36) ccw
  line L38 (-6.5846, 23.9988) -> (-32.0012, 49.4154)
  arc A22 (-29.5812, 51.2381) -> (-32.0012, 49.4154) centre (-20, 36) ccw
  arc A23 (-43.8553, 41.4828) -> (-55.5172, 53.1447) centre (-61, 36) ccw
  line L39 (-43.8553, 41.4828) -> (-55.5172, 53.1447)
  line L40 (-74.4154, 48.0012) -> (-48.9988, 22.5846)
  arc A24 (-51.4188, 20.7619) -> (-48.9988, 22.5846) centre (-61, 36) ccw
  line L41 (-51.4188, 20.7619) -> (-76.2381, 45.5812)
  arc A25 (-74.4154, 48.0012) -> (-76.2381, 45.5812) centre (-61, 36) ccw
  circle A26 centre (-77, 52) radius 2
  circle A27 centre (-4, 52) radius 2
  circle A28 centre (-40.5, 21) radius 2
  line L42 (-37.1447, 30.5172) -> (-25.4828, 18.8553)
  arc A29 (-37.1447, 30.5172) -> (-25.4828, 18.8553) centre (-20, 36) ccw
  line L43 (-78.1447, 30.5172) -> (-66.4828, 18.8553)
  arc A30 (-78.1447, 30.5172) -> (-66.4828, 18.8553) centre (-61, 36) ccw
  circle A31 centre (-40.5, 21) radius 5
  line L44 (2, 47) -> (-5.7522, 47)
  line L45 (-9, 56) -> (-9, 50.2478)
  line L46 (-74.4154, 48.0012) -> (-73.0012, 49.4154)
  line L47 (-75.2478, 47) -> (-83, 47)
  line L48 (-72, 50.2478) -> (-72, 56)
  dimension "d221" = 10
  dimension "d222" = 5
  dimension "d223" = 5
  dimension "d225" = 5
  dimension "d226" = 5
  constraint concentric A28 A31
  constraint coincident L14 L44.start
  constraint coincident A10 L44.end
  constraint perpendicular L14 L44
  constraint coincident L15 L45.start
  constraint coincident A10 L45.end
  constraint perpendicular L15 L45
  constraint coincident L40.start A25.start
  constraint coincident L28.end A12.end
  constraint coincident A25 L47.start
  constraint coincident L0 L47.end
  constraint perpendicular L0 L47
  constraint coincident A12 L48.start
  constraint coincident L15 L48.end
  constraint perpendicular L15 L48
  measures "d221" diameter of A31
  measures "d222" vertical distance of A27.centre L44.end
  measures "d223" horizontal distance of A27.centre L45.end
  measures "d225" vertical distance of A26.centre L47.start
  measures "d226" horizontal distance of A26.centre L48.start
extrude "Extrusion42" add sketch "Skizze31" along normal blind 3 contours L0 L15 A12 A25 L46 L47 L48 | L14 L15 A10 L44 L45 | A31 bodies 3
extrude "Extrusion43" cut sketch "Skizze30" against normal blind 20 contours L0 L18 L19 L20 L21 | L4 L14 L15 L16 L17 bodies 3
sketch "Skizze32" plane through (0, 0, 0) normal (0, 0, 1) x (1, 0, 0)
  line L0 (-4, -8.5) -> (0, -8.5)
  line L1 (0, -8.5) -> (0, -7)
  line L2 (0, -7) -> (-4, -7)
  line L3 (-4, -7) -> (-4, -8.5)
  line L4 (85, -7) -> (81, -7)
  line L5 (81, -7) -> (81, -8.5)
  line L6 (81, -8.5) -> (85, -8.5)
  line L7 (85, -8.5) -> (85, -7)
  point P0 (-5, -6)
  point P1 (86, -6)
  dimension "d247" = 4
  dimension "d248" = 1.5
  dimension "d249" = 1
  dimension "d250" = 1
  dimension "d251" = 4
  dimension "d252" = 1.5
  dimension "d254" = 1
  dimension "d255" = 1
  constraint horizontal L0
  constraint vertical L1
  constraint horizontal L2
  constraint vertical L3
  constraint horizontal L4
  constraint vertical L5
  constraint horizontal L6
  constraint vertical L7
  measures "d247" distance of L1.end L2.end
  measures "d248" distance of L0.start L2.end
  measures "d249" horizontal distance of L0.start P0
  measures "d250" vertical distance of L2.end P0
  measures "d251" distance of L4.start L4.end
  measures "d252" distance of L4.start L6.end
  measures "d254" horizontal distance of L6.end P1
  measures "d255" vertical distance of L4.start P1
extrude "Extrusion44" cut sketch "Skizze32" along normal blind 70 bodies 4
sketch "Skizze33" plane through (0, -6, 0) normal (0, 1, 0) x (-1, 0, 0)
  line L0 (5, 37) -> (5, 40)
  line L1 (5, 40) -> (-86, 40)
  line L2 (-86, 40) -> (-86, 37)
  line L3 (-86, 37) -> (5, 37)
  line L4 (-85, 38.25) -> (-81, 38.25)
  line L5 (-81, 38.25) -> (-81, 36.25)
  line L6 (-81, 36.25) -> (-85, 36.25)
  line L7 (-85, 36.25) -> (-85, 38.25)
  line L8 (4, 38.25) -> (0, 38.25)
  line L9 (0, 38.25) -> (0, 36.25)
  line L10 (0, 36.25) -> (4, 36.25)
  line L11 (4, 36.25) -> (4, 38.25)
  dimension "d266" = 1.75
  dimension "d267" = 1
  dimension "d268" = 2
  dimension "d269" = 4
  dimension "d270" = 1
  dimension "d272" = 1.75
  dimension "d273" = 2
  dimension "d274" = 4
  constraint horizontal L4
  constraint vertical L5
  constraint horizontal L6
  constraint vertical L7
  constraint horizontal L8
  constraint vertical L9
  constraint horizontal L10
  constraint vertical L11
  measures "d266" vertical distance of L1.end L4.start
  measures "d267" horizontal distance of L1.end L4.start
  measures "d268" distance of L4.start L6.end
  measures "d269" distance of L4.start L4.end
  measures "d270" horizontal distance of L0.end L8.start
  measures "d272" vertical distance of L0.end L8.start
  measures "d273" distance of L8.start L10.end
  measures "d274" distance of L8.start L8.end
extrude "Extrusion46" cut sketch "Skizze33" against normal blind 2.5 contours L3 L9 L10 L11 | L3 L8 L9 L11 | L3 L5 L6 L7 | L3 L4 L5 L7 bodies 4
fillet "Abrundung2" radius 0.5 2 edges at (-2, -7, 38.25) (83, -7, 38.25) on bodies 4
fillet "Abrundung3" radius 0.5 2 edges at (-2, 0, 38.5) (83, 0, 38.5) on bodies 3
hidden bodies 1 2
named bodies: "Lüfter", "Lüfter (1)", "Lüfter Halterung", "Lüfter Deckel"
